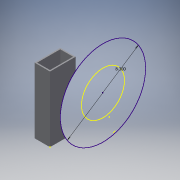
# Autodesk Inventor part: Frame Croner Opposite
Saved by Autodesk Inventor 2017 (Build 210142000, 142)
## iProperties
Created: 2019-01-17
Part Number: Frame Croner Opposite
Material: Generic
Document SubType Name: Modeling
Designer: S346795925
Density: 1 g/cm^3
Appearance: Default
Author: S346795925
Autodesk Inventor part; units mm, degrees
ref_plane "YZ Plane" through (0, 0, 0) normal (1, 0, 0) x (0, 1, 0)
ref_plane "XZ Plane" through (0, 0, 0) normal (0, 1, 0) x (-1, 0, 0)
ref_plane "XY Plane" through (0, 0, 0) normal (0, 0, 1) x (1, 0, 0)
sketch "Sketch1" plane through (0, 0, 0) normal (0, 1, 0) x (-1, 0, 0)
  line L0 (0, 0) -> (-38.1, 0)
  line L1 (-38.1, 0) -> (-38.1, -63.5)
  line L2 (-38.1, -63.5) -> (0, -63.5)
  line L3 (0, -63.5) -> (0, 0)
  line L4 (-3.175, -3.175) -> (-34.925, -3.175)
  line L5 (-34.925, -3.175) -> (-34.925, -60.325)
  line L6 (-34.925, -60.325) -> (-3.175, -60.325)
  line L7 (-3.175, -60.325) -> (-3.175, -3.175)
  dimension "d0" = 38.1
  dimension "d1" = 63.5
  dimension "d2" = 3.175
  constraints: 16 end point, 4 parallel, 2 perpendicular, 1 horizontal, 3 other
  measures "d0" distance of L2.end L1.end
  measures "d1" distance of L1.end L0.end
  measures "d2" distance between parallel lines of L3 L7
extrude "Extrusion1" add sketch "Sketch1" along normal blind 161.925
sketch "Sketch4" plane through (38.1, 0, 0) normal (1, 0, 0) x (0, 0, -1)
  circle A0 centre (130.683, 51.181) radius 105.41
  circle A1 centre (130.683, 51.181) radius 53.1813 projected
  ellipse E0 centre (147.1552, -8.6501) end of major axis (154.6171, -47.0051) minor radius 29.2764 (155.9011, -46.7151) -> (160.9598, -44.7271) ccw projected
  point P0 (0, 0)
  dimension "d14" = 210.82
  constraints: 1 centre point, 1 coincident, 1 other
  measures "d14" diameter of A0
extrude "Extrusion5" cut sketch "Sketch4" against normal blind 60.325 contours A0 | A1
body "Solid1"
